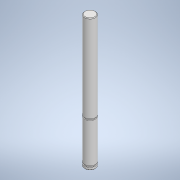
# Autodesk Inventor part: SHAFT
Saved by Autodesk Inventor 2022 (Build 260153000, 153)
## iProperties
Created: 2022-07-28
Part Number: SHAFT
Material: Generic
Document SubType Name: Modeling
Designer: Nathan Cai
Density: 1 g/cm^3
Appearance: Default
Author: Nathan Cai
Autodesk Inventor part; units mm, degrees
ref_plane "YZ Plane" through (0, 0, 0) normal (1, 0, 0) x (0, 1, 0)
ref_plane "XZ Plane" through (0, 0, 0) normal (0, 1, 0) x (-1, 0, 0)
ref_plane "XY Plane" through (0, 0, 0) normal (0, 0, 1) x (1, 0, 0)
sketch "Sketch2" plane through (0, 0, 0) normal (0, 0, 1) x (1, 0, 0)
  line L0 (0, 0) -> (2, 0)
  line L1 (2, 0) -> (2, 48.75)
  line L2 (2, 48.75) -> (0, 48.75)
  line L3 (0, 48.75) -> (0, 0)
  line L4 (2, 1) -> (1.75, 1)
  line L5 (1.75, 1) -> (1.75, 1.5)
  line L6 (1.75, 1.5) -> (2, 1.5)
  line L7 (2, 1.5) -> (2, 1)
  line L8 (2, 16) -> (1.75, 16)
  line L9 (1.75, 16) -> (1.75, 16.5)
  line L10 (1.75, 16.5) -> (2, 16.5)
  line L11 (2, 16.5) -> (2, 16)
  dimension "d3" = 2
  dimension "d4" = 48.75
  dimension "d5" = 1
  dimension "d6" = 0.5
  dimension "d7" = 0.25
  dimension "d8" = 16
  dimension "d9" = 0.5
  dimension "d10" = 0.25
  constraints: 24 end point, 6 parallel, 3 horizontal, 3 perpendicular, 2 point on line
  measures "d3" distance of L2.end L1.end
  measures "d4" distance of L1.end L0.end
  measures "d5" distance between parallel lines of L0 L4
  measures "d6" distance between parallel lines of L4 L6
  measures "d7" distance between parallel lines of L1 L5
  measures "d8" distance between parallel lines of L0 L8
  measures "d9" distance between parallel lines of L8 L10
  measures "d10" distance between parallel lines of L1 L9
revolve "Revolution1" add sketch "Sketch2" angle 360 about axis through (0, 48.75, 0) along (0, -1, 0) contours L3 L2 L1 L10 L9 L8 L6 L5 L4 L0
chamfer "Chamfer1" distance 0.25 angle 45 2 edges at (-2, 48.75, 0) (-2, 0, 0)
body "Solid2"
